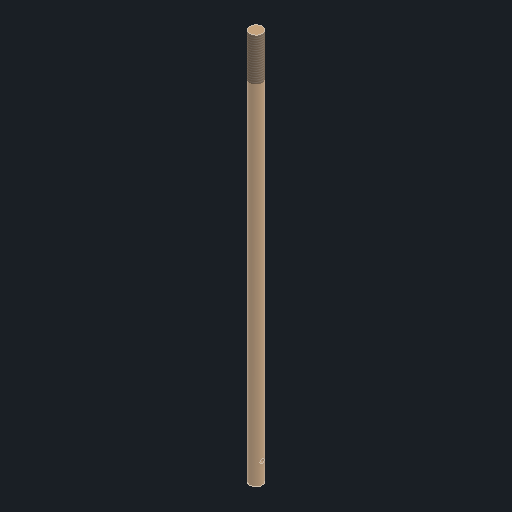
# Autodesk Inventor part: Pendulum Arm
Saved by Autodesk Inventor 2027.1 (Build 311270010, 270A)
## iProperties
Created: 2025-09-16
Part Number: Pendulum Arm
Material: Stainless Steel
Document SubType Name: Modeling
Designer: SD
Density: 8 g/cm^3
Appearance: Brindle
Mass: 5.77044 g
Surface Area: 8.80652 cm^2
Volume: 0.650264 cm^3
Project: Automatic Tea Steeping mechanism
Length: 92.000 mm
BOM-Mass: 0.00577
BOM-Area: 0.001
Procurement: Fabricate - 1st round
Build Stage: 1
Preferred Material: 303 Stainless Steel
Author: SD
Title: Pendulum Arm
Autodesk Inventor part; units mm, degrees
ref_plane "YZ Plane" through (0, 0, 0) normal (1, 0, 0) x (0, 1, 0)
ref_plane "XZ Plane" through (0, 0, 0) normal (0, 1, 0) x (-1, 0, 0)
ref_plane "XY Plane" through (0, 0, 0) normal (0, 0, 1) x (1, 0, 0)
sketch "Sketch1" plane through (0, 0, 0) normal (0, 1, 0) x (-1, 0, 0)
  circle A0 centre (0, 0) radius 1.5
  dimension "Diameter" = 3
  constraints: 1 centre point, 1 coincident
  measures "Diameter" diameter of A0
extrude "Extrusion1" add sketch "Sketch1" along normal mid plane 92
thread "Thread1" size "M3x0.5" class "6g" standard "ANSI Metric M Profile" length 10
chamfer "Chamfer1" distance 0.1 angle 45 1 edges at (1.5, -46, 0)
sketch "Sketch2" plane through (0, 0, 0) normal (1, 0, 0) x (0, 1, 0)
  line L0 (-46, -1.4) -> (-46, 1.4) projected
  point P0 (0, 0)
  point P1 (-41, 0)
  dimension "d8" = 5
  constraints: 1 horizontal alignment
  measures "d8" distance from line of point (-41, 0) L0
hole "Hole1" at (0, -41, 0) direction (-1, 0, 0) diameter 1 end through all both
body "Solid1"
